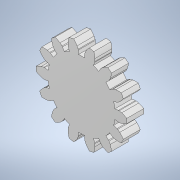
# Autodesk Inventor part: 二段多段部分歯数14
Saved by Autodesk Inventor 2022.2 (Build 262287030, 287C)
## iProperties
Created: 2022-02-22
Part Number: 二段多段部分歯数14
Material: Aluminum 2014-T6
Document SubType Name: Modeling
Designer: acps
Density: 2.78927 g/cm^3
Appearance: Satin
Author: acps
Autodesk Inventor part; units mm, degrees
ref_plane "YZ Plane" through (0, 0, 0) normal (1, 0, 0) x (0, 1, 0)
ref_plane "XZ Plane" through (0, 0, 0) normal (0, 1, 0) x (-1, 0, 0)
ref_plane "XY Plane" through (0, 0, 0) normal (0, 0, 1) x (1, 0, 0)
sketch "Sketch1" plane through (0, 0, 0) normal (0, 0, 1) x (1, 0, 0)
  arc A0 (0.6013, 6.6871) -> (0.5709, 6.553) centre (1.319, 6.4537) ccw
  arc A1 (0.7877, 7.1092) -> (0.6013, 6.6871) centre (2.5969, 6.0581) ccw
  arc A2 (1.382, 7.8797) -> (0.7877, 7.1092) centre (3.9753, 5.2649) ccw
  arc A3 (-2.3597, 6.2858) -> (-2.3289, 6.1518) centre (-1.6118, 6.3868) ccw
  arc A4 (-2.3755, 6.7383) -> (-2.3597, 6.2858) centre (-0.2888, 6.5849) ccw
  arc A5 (-2.1737, 7.699) -> (-2.3755, 6.7383) centre (1.2972, 6.4683) ccw
  arc A6 (-4.8533, 4.6395) -> (-4.7674, 4.5321) centre (-4.2233, 5.055) ccw
  arc A7 (-5.0639, 5.0403) -> (-4.8533, 4.6395) centre (-3.1173, 5.8075) ccw
  arc A8 (-5.2989, 5.9934) -> (-5.0639, 5.0403) centre (-1.6377, 6.3906) ccw
  arc A9 (-6.3857, 2.0743) -> (-6.2617, 2.0147) centre (-5.9984, 2.722) ccw
  arc A10 (-6.7557, 2.3499) -> (-6.3857, 2.0743) centre (-5.3284, 3.8798) ccw
  arc A11 (-7.3746, 3.1008) -> (-6.7557, 2.3499) centre (-4.2483, 5.0472) ccw
  arc A12 (-6.6533, -0.9018) -> (-6.5158, -0.9016) centre (-6.5853, -0.1502) ccw
  arc A13 (-7.1062, -0.814) -> (-6.6533, -0.9018) centre (-6.4841, 1.1837) ccw
  arc A14 (-7.9897, -0.406) -> (-7.1062, -0.814) centre (-6.0175, 2.7041) ccw
  arc A15 (-5.6031, -3.6992) -> (-5.4793, -3.6394) centre (-5.868, -2.9926) ccw
  arc A16 (-6.0493, -3.8167) -> (-5.6031, -3.6992) centre (-6.3556, -1.7469) ccw
  arc A17 (-7.0223, -3.8324) -> (-6.0493, -3.8167) centre (-6.5948, -0.1746) ccw
  arc A18 (-3.4432, -5.764) -> (-3.3576, -5.6564) centre (-3.9885, -5.2423) ccw
  arc A19 (-3.7942, -6.0634) -> (-3.4432, -5.764) centre (-4.9682, -4.3315) ccw
  arc A20 (-4.6641, -6.4997) -> (-3.7942, -6.0634) centre (-5.866, -3.0187) ccw
  arc A21 (-0.6013, -6.6871) -> (-0.5709, -6.553) centre (-1.319, -6.4537) ccw
  arc A22 (-0.7877, -7.1092) -> (-0.6013, -6.6871) centre (-2.5969, -6.0581) ccw
  arc A23 (-1.382, -7.8797) -> (-0.7877, -7.1092) centre (-3.9753, -5.2649) ccw
  arc A24 (2.3597, -6.2858) -> (2.3289, -6.1518) centre (1.6118, -6.3868) ccw
  arc A25 (2.3749, -6.7469) -> (2.3597, -6.2858) centre (0.2888, -6.5849) ccw
  arc A26 (2.1737, -7.699) -> (2.3749, -6.7469) centre (-1.2972, -6.4683) ccw
  arc A27 (4.8533, -4.6395) -> (4.7674, -4.5321) centre (4.2233, -5.055) ccw
  arc A28 (5.0671, -5.0483) -> (4.8533, -4.6395) centre (3.1173, -5.8075) ccw
  arc A29 (5.2989, -5.9934) -> (5.0671, -5.0483) centre (1.6377, -6.3906) ccw
  arc A30 (6.3857, -2.0743) -> (6.2617, -2.0147) centre (5.9984, -2.722) ccw
  arc A31 (6.7557, -2.3499) -> (6.3857, -2.0743) centre (5.3284, -3.8798) ccw
  arc A32 (7.3746, -3.1008) -> (6.7557, -2.3499) centre (4.2483, -5.0472) ccw
  arc A33 (6.6533, 0.9018) -> (6.5158, 0.9016) centre (6.5853, 0.1502) ccw
  arc A34 (7.1062, 0.814) -> (6.6533, 0.9018) centre (6.4841, -1.1837) ccw
  arc A35 (7.9897, 0.406) -> (7.1062, 0.814) centre (6.0175, -2.7041) ccw
  arc A36 (5.6031, 3.6992) -> (5.4793, 3.6394) centre (5.868, 2.9926) ccw
  arc A37 (6.0408, 3.8154) -> (5.6031, 3.6992) centre (6.3556, 1.7469) ccw
  arc A38 (7.0223, 3.8324) -> (6.0408, 3.8154) centre (6.5948, 0.1746) ccw
  arc A39 (3.4432, 5.764) -> (3.3576, 5.6564) centre (3.9885, 5.2423) ccw
  arc A40 (3.7942, 6.0634) -> (3.4432, 5.764) centre (4.9682, 4.3315) ccw
  arc A41 (4.6641, 6.4997) -> (3.7942, 6.0634) centre (5.866, 3.0187) ccw
  arc A42 (-0.5709, 6.553) -> (-0.6013, 6.6871) centre (-1.319, 6.4537) ccw
  arc A43 (-0.6013, 6.6871) -> (-0.7834, 7.1017) centre (-2.5969, 6.0581) ccw
  arc A44 (-0.7834, 7.1017) -> (-1.382, 7.8797) centre (-3.9753, 5.2649) ccw
  arc A45 (-3.3576, 5.6564) -> (-3.4432, 5.764) centre (-3.9885, 5.2423) ccw
  arc A46 (-3.4432, 5.764) -> (-3.7942, 6.0634) centre (-4.9682, 4.3315) ccw
  arc A47 (-3.7942, 6.0634) -> (-4.6641, 6.4997) centre (-5.866, 3.0187) ccw
  arc A48 (-5.4793, 3.6394) -> (-5.6031, 3.6992) centre (-5.868, 2.9926) ccw
  arc A49 (-5.6031, 3.6992) -> (-6.0493, 3.8167) centre (-6.3556, 1.7469) ccw
  arc A50 (-6.0493, 3.8167) -> (-7.0223, 3.8324) centre (-6.5948, 0.1746) ccw
  arc A51 (-6.5158, 0.9016) -> (-6.6533, 0.9018) centre (-6.5853, 0.1502) ccw
  arc A52 (-6.6533, 0.9018) -> (-7.1062, 0.814) centre (-6.4841, -1.1837) ccw
  arc A53 (-7.1062, 0.814) -> (-7.9897, 0.406) centre (-6.0175, -2.7041) ccw
  arc A54 (-6.2617, -2.0147) -> (-6.3857, -2.0743) centre (-5.9984, -2.722) ccw
  arc A55 (-6.3857, -2.0743) -> (-6.7557, -2.3499) centre (-5.3284, -3.8798) ccw
  arc A56 (-6.7557, -2.3499) -> (-7.3746, -3.1008) centre (-4.2483, -5.0472) ccw
  arc A57 (-4.7674, -4.5321) -> (-4.8533, -4.6395) centre (-4.2233, -5.055) ccw
  arc A58 (-4.8533, -4.6395) -> (-5.0671, -5.0483) centre (-3.1173, -5.8075) ccw
  arc A59 (-5.0671, -5.0483) -> (-5.2989, -5.9934) centre (-1.6377, -6.3906) ccw
  arc A60 (-2.3289, -6.1518) -> (-2.3597, -6.2858) centre (-1.6118, -6.3868) ccw
  arc A61 (-2.3597, -6.2858) -> (-2.3749, -6.7469) centre (-0.2888, -6.5849) ccw
  arc A62 (-2.3749, -6.7469) -> (-2.1737, -7.699) centre (1.2972, -6.4683) ccw
  arc A63 (0.5709, -6.553) -> (0.6013, -6.6871) centre (1.319, -6.4537) ccw
  arc A64 (0.6013, -6.6871) -> (0.7877, -7.1092) centre (2.5969, -6.0581) ccw
  arc A65 (0.7877, -7.1092) -> (1.382, -7.8797) centre (3.9753, -5.2649) ccw
  arc A66 (3.3576, -5.6564) -> (3.4432, -5.764) centre (3.9885, -5.2423) ccw
  arc A67 (3.4432, -5.764) -> (3.7942, -6.0634) centre (4.9682, -4.3315) ccw
  arc A68 (3.7942, -6.0634) -> (4.6641, -6.4997) centre (5.866, -3.0187) ccw
  arc A69 (5.4793, -3.6394) -> (5.6031, -3.6992) centre (5.868, -2.9926) ccw
  arc A70 (5.6031, -3.6992) -> (6.0493, -3.8167) centre (6.3556, -1.7469) ccw
  arc A71 (6.0493, -3.8167) -> (7.0223, -3.8324) centre (6.5948, -0.1746) ccw
  arc A72 (6.5158, -0.9016) -> (6.6533, -0.9018) centre (6.5853, -0.1502) ccw
  arc A73 (6.6533, -0.9018) -> (7.1062, -0.814) centre (6.4841, 1.1837) ccw
  arc A74 (7.1062, -0.814) -> (7.9897, -0.406) centre (6.0175, 2.7041) ccw
  arc A75 (6.2617, 2.0147) -> (6.3857, 2.0743) centre (5.9984, 2.722) ccw
  arc A76 (6.3857, 2.0743) -> (6.7557, 2.3499) centre (5.3284, 3.8798) ccw
  arc A77 (6.7557, 2.3499) -> (7.3746, 3.1008) centre (4.2483, 5.0472) ccw
  arc A78 (4.7674, 4.5321) -> (4.8533, 4.6395) centre (4.2233, 5.055) ccw
  arc A79 (4.8533, 4.6395) -> (5.0671, 5.0483) centre (3.1173, 5.8075) ccw
  arc A80 (5.0671, 5.0483) -> (5.2989, 5.9934) centre (1.6377, 6.3906) ccw
  arc A81 (2.3289, 6.1518) -> (2.3597, 6.2858) centre (1.6118, 6.3868) ccw
  arc A82 (2.3597, 6.2858) -> (2.3749, 6.7469) centre (0.2888, 6.5849) ccw
  arc A83 (2.3749, 6.7469) -> (2.1737, 7.699) centre (-1.2972, 6.4683) ccw
  arc A84 (0.5164, 5.9276) -> (-0.5164, 5.9275) centre (0, 0) ccw
  arc A85 (-2.1066, 5.5646) -> (-3.0371, 5.1165) centre (0, 0) ccw
  arc A86 (-4.3124, 4.0995) -> (-4.9563, 3.292) centre (0, 0) ccw
  arc A87 (-5.664, 1.8224) -> (-5.8938, 0.8156) centre (0, 0) ccw
  arc A88 (-5.8938, -0.8156) -> (-5.664, -1.8224) centre (0, 0) ccw
  arc A89 (-4.9563, -3.292) -> (-4.3124, -4.0995) centre (0, 0) ccw
  arc A90 (-3.0371, -5.1165) -> (-2.1066, -5.5646) centre (0, 0) ccw
  arc A91 (-0.5164, -5.9276) -> (0.5164, -5.9276) centre (0, 0) ccw
  arc A92 (2.1066, -5.5646) -> (3.0371, -5.1165) centre (0, 0) ccw
  arc A93 (4.3124, -4.0995) -> (4.9563, -3.292) centre (0, 0) ccw
  arc A94 (5.664, -1.8224) -> (5.8938, -0.8156) centre (0, 0) ccw
  arc A95 (5.8938, 0.8156) -> (5.664, 1.8224) centre (0, 0) ccw
  arc A96 (4.9563, 3.292) -> (4.3124, 4.0995) centre (0, 0) ccw
  arc A97 (3.0371, 5.1165) -> (2.1066, 5.5646) centre (0, 0) ccw
  arc A98 (-1.382, 7.8797) -> (-2.1737, 7.699) centre (0, 0) ccw
  arc A99 (-4.6641, 6.4997) -> (-5.2989, 5.9934) centre (0, 0) ccw
  arc A100 (-7.0223, 3.8324) -> (-7.3746, 3.1008) centre (0, 0) ccw
  arc A101 (-7.9897, 0.406) -> (-7.9897, -0.406) centre (0, 0) ccw
  arc A102 (-7.3746, -3.1008) -> (-7.0223, -3.8324) centre (0, 0) ccw
  arc A103 (-5.2989, -5.9934) -> (-4.6641, -6.4997) centre (0, 0) ccw
  arc A104 (-2.1737, -7.699) -> (-1.382, -7.8797) centre (0, 0) ccw
  arc A105 (1.382, -7.8797) -> (2.1737, -7.699) centre (0, 0) ccw
  arc A106 (4.6641, -6.4997) -> (5.2989, -5.9934) centre (0, 0) ccw
  arc A107 (7.0223, -3.8324) -> (7.3746, -3.1008) centre (0, 0) ccw
  arc A108 (7.9897, -0.406) -> (7.9897, 0.406) centre (0, 0) ccw
  arc A109 (7.3746, 3.1008) -> (7.0223, 3.8324) centre (0, 0) ccw
  arc A110 (5.2989, 5.9934) -> (4.6641, 6.4997) centre (0, 0) ccw
  arc A111 (2.1737, 7.699) -> (1.382, 7.8797) centre (0, 0) ccw
  line L0 (0.5164, 5.9276) -> (0.5709, 6.553)
  line L1 (-2.1066, 5.5646) -> (-2.3289, 6.1518)
  line L2 (-4.3124, 4.0995) -> (-4.7674, 4.5321)
  line L3 (-5.664, 1.8224) -> (-6.2617, 2.0147)
  line L4 (-5.8938, -0.8156) -> (-6.5158, -0.9016)
  line L5 (-4.9563, -3.292) -> (-5.4793, -3.6394)
  line L6 (-3.0371, -5.1165) -> (-3.3576, -5.6564)
  line L7 (-0.5164, -5.9276) -> (-0.5709, -6.553)
  line L8 (2.1066, -5.5646) -> (2.3289, -6.1518)
  line L9 (4.3124, -4.0995) -> (4.7674, -4.5321)
  line L10 (5.664, -1.8224) -> (6.2617, -2.0147)
  line L11 (5.8938, 0.8156) -> (6.5158, 0.9016)
  line L12 (4.9563, 3.292) -> (5.4793, 3.6394)
  line L13 (3.0371, 5.1165) -> (3.3576, 5.6564)
  line L14 (-0.5164, 5.9275) -> (-0.5709, 6.553)
  line L15 (-3.0371, 5.1165) -> (-3.3576, 5.6564)
  line L16 (-4.9563, 3.292) -> (-5.4793, 3.6394)
  line L17 (-5.8938, 0.8156) -> (-6.5158, 0.9016)
  line L18 (-5.664, -1.8224) -> (-6.2617, -2.0147)
  line L19 (-4.3124, -4.0995) -> (-4.7674, -4.5321)
  line L20 (-2.1066, -5.5646) -> (-2.3289, -6.1518)
  line L21 (0.5164, -5.9276) -> (0.5709, -6.553)
  line L22 (3.0371, -5.1165) -> (3.3576, -5.6564)
  line L23 (4.9563, -3.292) -> (5.4793, -3.6394)
  line L24 (5.8938, -0.8156) -> (6.5158, -0.9016)
  line L25 (5.664, 1.8224) -> (6.2617, 2.0147)
  line L26 (4.3124, 4.0995) -> (4.7674, 4.5321)
  line L27 (2.1066, 5.5646) -> (2.3289, 6.1518)
  point P0 (0, 0)
  constraints: 168 point on circle, 84 centre point, 56 end point, 2 horizontal alignment, 2 vertical alignment, 80 other
extrude "Extrusion1" add sketch "Sketch1" against normal blind 3
body "Solid1"
